Autodesk Inventor part; units mm, degrees
(part 3 of 4)
sketch "All Together" plane through (0, 0, 1.8) normal (0, 0, 1) x (1, 0, 0)
  arc A0 (70.625, 11.2735) -> (71.75, 14.25) centre (67.25, 14.25) ccw projected
  line L0 (71.75, 14.25) -> (71.75, 43.95) projected
  arc A1 (71.75, 43.95) -> (70.625, 46.9265) centre (67.25, 43.95) ccw projected
  arc A2 (70.1483, 47.7318) -> (70.625, 46.9265) centre (72.5, 48.5801) ccw projected
  arc A3 (70.1483, 47.7318) -> (69.436, 47.9997) centre (69.678, 47.5622) ccw projected
  arc A4 (63.9168, 53.2778) -> (69.436, 47.9997) centre (67.5, 51.5) ccw projected
  arc A5 (63.9168, 53.2778) -> (63.4689, 54) centre (63.4689, 53.5) ccw projected
  line L1 (63.4689, 54) -> (-63.4689, 54) projected
  arc A6 (-63.4689, 54) -> (-63.9168, 53.2778) centre (-63.4689, 53.5) ccw projected
  arc A7 (-69.2778, 47.9168) -> (-63.9168, 53.2778) centre (-67.5, 51.5) ccw projected
  arc A8 (-69.2778, 47.9168) -> (-70, 47.4689) centre (-69.5, 47.4689) ccw projected
  line L2 (-70, 47.4689) -> (-70, 22.5) projected
  line L3 (-70, 22.5) -> (-54, 22.5) projected
  arc A9 (-51.5, 20) -> (-54, 22.5) centre (-54, 20) ccw projected
  line L4 (-51.5, 20) -> (-51.5, 17.8589) projected
  arc A10 (-51.5, 17.8589) -> (-50.8913, 16.5323) centre (-49.75, 17.8589) ccw projected
  arc A11 (-53.5, 9.5) -> (-50.8913, 16.5323) centre (-53.5, 13.5) ccw projected
  line L5 (-53.5, 9.5) -> (-68.5, 9.5) projected
  arc A12 (-70.1109, 9.8387) -> (-68.5, 9.5) centre (-68.5, 13.5) ccw projected
  arc A13 (-70, 9.1411) -> (-70.1109, 9.8387) centre (-72.25, 9.1411) ccw projected
  line L6 (-70, 9.1411) -> (-70, 3.5) projected
  line L7 (-70, 3.5) -> (-52.9019, 3.5) projected
  line L8 (-52.9019, 3.5) -> (-51.3142, 0.75) projected
  arc A14 (-51.3142, -2.75) -> (-51.3142, 0.75) centre (-54.3453, -1) ccw projected
  line L9 (-51.3142, -2.75) -> (-52.9019, -5.5) projected
  line L10 (-52.9019, -5.5) -> (-70, -5.5) projected
  line L11 (-70, -5.5) -> (-70, -10.5) projected
  arc A15 (-70.1419, -11.4865) -> (-70, -10.5) centre (-73.5, -10.5) ccw projected
  arc A16 (-54.6724, -28.431) -> (-70.1419, -11.4865) centre (-63, -20.5) ccw projected
  arc A17 (-54.6724, -28.431) -> (-55.5, -30.5) centre (-52.5, -30.5) ccw projected
  line L12 (-55.5, -30.5) -> (-55.5, -32.5) projected
  arc A18 (-58, -35) -> (-55.5, -32.5) centre (-58, -32.5) ccw projected
  line L13 (-58, -35) -> (-70, -35) projected
  line L14 (-70, -35) -> (-70, -37) projected
  line L15 (-70, -37) -> (-56.4793, -37) projected
  line L16 (-56.4793, -37) -> (-55.1802, -39.25) projected
  arc A19 (-55.1802, -41.75) -> (-55.1802, -39.25) centre (-57.3453, -40.5) ccw projected
  line L17 (-55.1802, -41.75) -> (-56.4793, -44) projected
  line L18 (-56.4793, -44) -> (-70, -44) projected
  line L19 (-70, -44) -> (-70, -47.4689) projected
  arc A20 (-70, -47.4689) -> (-69.2778, -47.9168) centre (-69.5, -47.4689) ccw projected
  arc A21 (-63.9168, -53.2778) -> (-69.2778, -47.9168) centre (-67.5, -51.5) ccw projected
  arc A22 (-63.9168, -53.2778) -> (-63.4689, -54) centre (-63.4689, -53.5) ccw projected
  line L20 (-63.4689, -54) -> (-47.5, -54) projected
  line L21 (-47.5, -54) -> (-47.5, -50) projected
  arc A23 (-45, -47.5) -> (-47.5, -50) centre (-45, -50) ccw projected
  line L22 (-45, -47.5) -> (24, -47.5) projected
  arc A24 (26.5, -50) -> (24, -47.5) centre (24, -50) ccw projected
  line L23 (26.5, -50) -> (26.5, -54) projected
  line L24 (26.5, -54) -> (63.4689, -54) projected
  arc A25 (63.4689, -54) -> (63.9168, -53.2778) centre (63.4689, -53.5) ccw projected
  arc A26 (69.2778, -47.9168) -> (63.9168, -53.2778) centre (67.5, -51.5) ccw projected
  arc A27 (69.2778, -47.9168) -> (70, -47.4689) centre (69.5, -47.4689) ccw projected
  line L25 (70, -47.4689) -> (70, -44) projected
  line L26 (70, -44) -> (56.366, -44) projected
  line L27 (56.366, -44) -> (58.0981, -41) projected
  arc A28 (58.0981, -41) -> (58.0981, -40) centre (57.2321, -40.5) ccw projected
  line L28 (58.0981, -40) -> (56.366, -37) projected
  line L29 (56.366, -37) -> (70, -37) projected
  line L30 (70, -37) -> (70, -30.5) projected
  arc A29 (70.1419, -29.5135) -> (70, -30.5) centre (73.5, -30.5) ccw projected
  arc A30 (54.6724, -12.569) -> (70.1419, -29.5135) centre (63, -20.5) ccw projected
  arc A31 (54.6724, -12.569) -> (55.5, -10.5) centre (52.5, -10.5) ccw projected
  line L31 (55.5, -10.5) -> (55.5, -8.5) projected
  arc A32 (58, -6) -> (55.5, -8.5) centre (58, -8.5) ccw projected
  line L32 (58, -6) -> (70, -6) projected
  line L33 (70, -6) -> (70, 9.6199) projected
  arc A33 (70.625, 11.2735) -> (70, 9.6199) centre (72.5, 9.6199) ccw projected
  line L34 (36.5, -14.0193) -> (36.5, -6) projected
  arc A34 (47.5, -6) -> (36.5, -6) centre (42, -6) ccw projected
  line L35 (47.5, -6) -> (47.5, -14.0193) projected
  arc A35 (49.5, -24.5) -> (47.5, -14.0193) centre (42, -20.5) ccw projected
  line L36 (49.5, -24.5) -> (49.5, -33.5) projected
  arc A36 (47, -36) -> (49.5, -33.5) centre (47, -33.5) ccw projected
  line L37 (47, -36) -> (37, -36) projected
  arc A37 (34.5, -33.5) -> (37, -36) centre (37, -33.5) ccw projected
  line L38 (34.5, -33.5) -> (34.5, -24.5) projected
  arc A38 (34.3389, -16.8179) -> (34.5, -24.5) centre (42, -20.5) ccw projected
  arc A39 (28.6611, -16.8179) -> (34.3389, -16.8179) centre (31.5, -14) ccw projected
  arc A40 (26.5, -26.9807) -> (28.6611, -16.8179) centre (21, -20.5) ccw projected
  line L39 (26.5, -26.9807) -> (26.5, -33.5) projected
  arc A41 (24, -36) -> (26.5, -33.5) centre (24, -33.5) ccw projected
  line L40 (24, -36) -> (18, -36) projected
  arc A42 (15.5, -33.5) -> (18, -36) centre (18, -33.5) ccw projected
  line L41 (15.5, -33.5) -> (15.5, -26.9807) projected
  arc A43 (13.3389, -16.8179) -> (15.5, -26.9807) centre (21, -20.5) ccw projected
  arc A44 (7.6611, -16.8179) -> (13.3389, -16.8179) centre (10.5, -14) ccw projected
  arc A45 (5.5, -26.9807) -> (7.6611, -16.8179) centre (0, -20.5) ccw projected
  line L42 (5.5, -26.9807) -> (5.5, -33.5) projected
  arc A46 (3, -36) -> (5.5, -33.5) centre (3, -33.5) ccw projected
  line L43 (3, -36) -> (-3, -36) projected
  arc A47 (-5.5, -33.5) -> (-3, -36) centre (-3, -33.5) ccw projected
  line L44 (-5.5, -33.5) -> (-5.5, -26.9807) projected
  arc A48 (-7.6611, -16.8179) -> (-5.5, -26.9807) centre (0, -20.5) ccw projected
  arc A49 (-13.3389, -16.8179) -> (-7.6611, -16.8179) centre (-10.5, -14) ccw projected
  arc A50 (-15.5, -26.9807) -> (-13.3389, -16.8179) centre (-21, -20.5) ccw projected
  line L45 (-15.5, -26.9807) -> (-15.5, -33.5) projected
  arc A51 (-18, -36) -> (-15.5, -33.5) centre (-18, -33.5) ccw projected
  line L46 (-18, -36) -> (-24, -36) projected
  arc A52 (-26.5, -33.5) -> (-24, -36) centre (-24, -33.5) ccw projected
  line L47 (-26.5, -33.5) -> (-26.5, -26.9807) projected
  arc A53 (-28.6611, -16.8179) -> (-26.5, -26.9807) centre (-21, -20.5) ccw projected
  arc A54 (-34.3389, -16.8179) -> (-28.6611, -16.8179) centre (-31.5, -14) ccw projected
  arc A55 (-36.5, -26.9807) -> (-34.3389, -16.8179) centre (-42, -20.5) ccw projected
  line L48 (-36.5, -26.9807) -> (-36.5, -33.5) projected
  arc A56 (-39, -36) -> (-36.5, -33.5) centre (-39, -33.5) ccw projected
  line L49 (-39, -36) -> (-45, -36) projected
  arc A57 (-47.5, -33.5) -> (-45, -36) centre (-45, -33.5) ccw projected
  line L50 (-47.5, -33.5) -> (-47.5, -26.9807) projected
  arc A58 (-47.5, -14.0193) -> (-47.5, -26.9807) centre (-42, -20.5) ccw projected
  line L51 (-47.5, -14.0193) -> (-47.5, -6) projected
  arc A59 (-36.5, -6) -> (-47.5, -6) centre (-42, -6) ccw projected
  line L52 (-36.5, -6) -> (-36.5, -14.0193) projected
  arc A60 (-35.2881, -15.2846) -> (-36.5, -14.0193) centre (-42, -20.5) ccw projected
  arc A61 (-27.7119, -15.2846) -> (-35.2881, -15.2846) centre (-31.5, -14) ccw projected
  arc A62 (-26.5, -14.0193) -> (-27.7119, -15.2846) centre (-21, -20.5) ccw projected
  line L53 (-26.5, -14.0193) -> (-26.5, -6) projected
  arc A63 (-15.5, -6) -> (-26.5, -6) centre (-21, -6) ccw projected
  line L54 (-15.5, -6) -> (-15.5, -14.0193) projected
  arc A64 (-14.2881, -15.2846) -> (-15.5, -14.0193) centre (-21, -20.5) ccw projected
  arc A65 (-6.7119, -15.2846) -> (-14.2881, -15.2846) centre (-10.5, -14) ccw projected
  arc A66 (-5.5, -14.0193) -> (-6.7119, -15.2846) centre (0, -20.5) ccw projected
  line L55 (-5.5, -14.0193) -> (-5.5, -6) projected
  arc A67 (5.5, -6) -> (-5.5, -6) centre (0, -6) ccw projected
  line L56 (5.5, -6) -> (5.5, -14.0193) projected
  arc A68 (6.7119, -15.2846) -> (5.5, -14.0193) centre (0, -20.5) ccw projected
  arc A69 (14.2881, -15.2846) -> (6.7119, -15.2846) centre (10.5, -14) ccw projected
  arc A70 (15.5, -14.0193) -> (14.2881, -15.2846) centre (21, -20.5) ccw projected
  line L57 (15.5, -14.0193) -> (15.5, -6) projected
  arc A71 (26.5, -6) -> (15.5, -6) centre (21, -6) ccw projected
  line L58 (26.5, -6) -> (26.5, -14.0193) projected
  arc A72 (27.7119, -15.2846) -> (26.5, -14.0193) centre (21, -20.5) ccw projected
  arc A73 (35.2881, -15.2846) -> (27.7119, -15.2846) centre (31.5, -14) ccw projected
  arc A74 (36.5, -14.0193) -> (35.2881, -15.2846) centre (42, -20.5) ccw projected
  circle A75 centre (35.75, 14.25) radius 3 projected
  line L59 (71, 39.1) -> (71, 22.1) projected
  arc A76 (67.5, 18.6) -> (71, 22.1) centre (67.5, 22.1) ccw projected
  line L60 (67.5, 18.6) -> (35.5, 18.6) projected
  arc A77 (32, 22.1) -> (35.5, 18.6) centre (35.5, 22.1) ccw projected
  line L61 (32, 22.1) -> (32, 39.1) projected
  arc A78 (33.4964, 41.9698) -> (32, 39.1) centre (35.5, 39.1) ccw projected
  arc A79 (38.4291, 42.6) -> (33.4964, 41.9698) centre (35.75, 43.95) ccw projected
  line L62 (38.4291, 42.6) -> (64.5709, 42.6) projected
  arc A80 (69.5036, 41.9698) -> (64.5709, 42.6) centre (67.25, 43.95) ccw projected
  arc A81 (71, 39.1) -> (69.5036, 41.9698) centre (67.5, 39.1) ccw projected
  circle A82 centre (67.25, 14.25) radius 3 projected
  circle A83 centre (-31.5, -14) radius 3.5 projected
  circle A84 centre (-31.5, -14) radius 1.6 projected
  circle A85 centre (-10.5, -14) radius 3.5 projected
  circle A86 centre (-10.5, -14) radius 1.6 projected
  circle A87 centre (10.5, -14) radius 3.5 projected
  circle A88 centre (10.5, -14) radius 1.6 projected
  circle A89 centre (31.5, -14) radius 3.5 projected
  circle A90 centre (31.5, -14) radius 1.6 projected
  line L63 (16, -6) -> (16, -14.255) projected
  arc A91 (26, -14.255) -> (16, -14.255) centre (21, -20.5) ccw projected
  line L64 (26, -14.255) -> (26, -6) projected
  arc A92 (26, -6) -> (16, -6) centre (21, -6) ccw projected
  circle A93 centre (21, -6) radius 2.75 projected
  line L65 (26, -33.5) -> (26, -26.745) projected
  arc A94 (16, -26.745) -> (26, -26.745) centre (21, -20.5) ccw projected
  line L66 (16, -26.745) -> (16, -33.5) projected
  arc A95 (16, -33.5) -> (18, -35.5) centre (18, -33.5) ccw projected
  line L67 (18, -35.5) -> (24, -35.5) projected
  arc A96 (24, -35.5) -> (26, -33.5) centre (24, -33.5) ccw projected
  line L68 (5, -33.5) -> (5, -26.745) projected
  arc A97 (-5, -26.745) -> (5, -26.745) centre (0, -20.5) ccw projected
  line L69 (-5, -26.745) -> (-5, -33.5) projected
  arc A98 (-5, -33.5) -> (-3, -35.5) centre (-3, -33.5) ccw projected
  line L70 (-3, -35.5) -> (3, -35.5) projected
  arc A99 (3, -35.5) -> (5, -33.5) centre (3, -33.5) ccw projected
  line L71 (-16, -33.5) -> (-16, -26.745) projected
  arc A100 (-26, -26.745) -> (-16, -26.745) centre (-21, -20.5) ccw projected
  line L72 (-26, -26.745) -> (-26, -33.5) projected
  arc A101 (-26, -33.5) -> (-24, -35.5) centre (-24, -33.5) ccw projected
  line L73 (-24, -35.5) -> (-18, -35.5) projected
  arc A102 (-18, -35.5) -> (-16, -33.5) centre (-18, -33.5) ccw projected
  line L74 (-37, -33.5) -> (-37, -26.745) projected
  arc A103 (-47, -26.745) -> (-37, -26.745) centre (-42, -20.5) ccw projected
  line L75 (-47, -26.745) -> (-47, -33.5) projected
  arc A104 (-47, -33.5) -> (-45, -35.5) centre (-45, -33.5) ccw projected
  line L76 (-45, -35.5) -> (-39, -35.5) projected
  arc A105 (-39, -35.5) -> (-37, -33.5) centre (-39, -33.5) ccw projected
  line L77 (-47, -6) -> (-47, -14.255) projected
  arc A106 (-37, -14.255) -> (-47, -14.255) centre (-42, -20.5) ccw projected
  line L78 (-37, -14.255) -> (-37, -6) projected
  arc A107 (-37, -6) -> (-47, -6) centre (-42, -6) ccw projected
  circle A108 centre (-42, -6) radius 2.75 projected
  line L79 (-26, -6) -> (-26, -14.255) projected
  arc A109 (-16, -14.255) -> (-26, -14.255) centre (-21, -20.5) ccw projected
  line L80 (-16, -14.255) -> (-16, -6) projected
  arc A110 (-16, -6) -> (-26, -6) centre (-21, -6) ccw projected
  circle A111 centre (-21, -6) radius 2.75 projected
  line L81 (-5, -6) -> (-5, -14.255) projected
  arc A112 (5, -14.255) -> (-5, -14.255) centre (0, -20.5) ccw projected
  line L82 (5, -14.255) -> (5, -6) projected
  arc A113 (5, -6) -> (-5, -6) centre (0, -6) ccw projected
  circle A114 centre (0, -6) radius 2.75 projected
  line L83 (38, -6) -> (38, -13.5718) projected
  arc A115 (46, -13.5718) -> (38, -13.5718) centre (42, -20.5) ccw projected
  line L84 (46, -13.5718) -> (46, -6) projected
  arc A116 (46, -6) -> (38, -6) centre (42, -6) ccw projected
  circle A117 centre (42, -6) radius 2.75 projected
  line L85 (37.5, -30) -> (37.5, -27.1144) projected
  arc A118 (35, -24.373) -> (37.5, -27.1144) centre (42, -20.5) ccw projected
  line L86 (35, -33.5) -> (35, -24.373) projected
  arc A119 (35, -33.5) -> (37, -35.5) centre (37, -33.5) ccw projected
  line L87 (47, -35.5) -> (37, -35.5) projected
  arc A120 (47, -35.5) -> (49, -33.5) centre (47, -33.5) ccw projected
  line L88 (49, -24.373) -> (49, -33.5) projected
  arc A121 (46.5, -27.1144) -> (49, -24.373) centre (42, -20.5) ccw projected
  line L89 (46.5, -27.1144) -> (46.5, -30) projected
  line L90 (46.5, -30) -> (46, -30) projected
  line L91 (46, -30) -> (46, -27.4282) projected
  arc A122 (38, -27.4282) -> (46, -27.4282) centre (42, -20.5) ccw projected
  line L92 (38, -27.4282) -> (38, -30) projected
  line L93 (38, -30) -> (37.5, -30) projected
  arc A123 (46.5, -6) -> (37.5, -6) centre (42, -6) ccw projected
  line L94 (37.5, -13.8856) -> (37.5, -6) projected
  arc A124 (38, -13.5718) -> (37.5, -13.8856) centre (42, -20.5) ccw projected
  line L95 (38, -6) -> (38, -13.5718) projected
  arc A125 (46, -6) -> (38, -6) centre (42, -6) ccw projected
  line L96 (46, -13.5718) -> (46, -6) projected
  arc A126 (46.5, -13.8856) -> (46, -13.5718) centre (42, -20.5) ccw projected
  line L97 (46.5, -6) -> (46.5, -13.8856) projected
  circle A127 centre (63, -20.5) radius 8 projected
  arc A128 (70, -10.5) -> (70.9655, -12.9138) centre (73.5, -10.5) ccw projected
  line L98 (70, -6.5) -> (70, -10.5) projected
  line L99 (58, -6.5) -> (70, -6.5) projected
  arc A129 (58, -6.5) -> (56, -8.5) centre (58, -8.5) ccw projected
  line L100 (56, -10.5) -> (56, -8.5) projected
  arc A130 (55.0345, -12.9138) -> (56, -10.5) centre (52.5, -10.5) ccw projected
  arc A131 (55.0345, -12.9138) -> (70.9655, -12.9138) centre (63, -20.5) ccw projected
  line L101 (-70.5, -37.5) -> (-70.5, -30.5) projected
  arc A132 (-70.5, -30.5) -> (-71.3276, -28.431) centre (-73.5, -30.5) ccw projected
  arc A133 (-71.3276, -12.569) -> (-71.3276, -28.431) centre (-63, -20.5) ccw projected
  arc A134 (-71.3276, -12.569) -> (-70.5, -10.5) centre (-73.5, -10.5) ccw projected
  line L102 (-70.5, -10.5) -> (-70.5, -5) projected
  line L103 (-53.1906, -5) -> (-70.5, -5) projected
  line L104 (-51.7472, -2.5) -> (-53.1906, -5) projected
  arc A135 (-51.7472, -2.5) -> (-51.7472, 0.5) centre (-54.3453, -1) ccw projected
  line L105 (-53.1906, 3) -> (-51.7472, 0.5) projected
  line L106 (-70.5, 3) -> (-53.1906, 3) projected
  line L107 (-70.5, 3) -> (-70.5, 9.1411) projected
  arc A136 (-70.5, 9.1411) -> (-71.1087, 10.4677) centre (-72.25, 9.1411) ccw projected
  arc A137 (-71.1087, 16.5323) -> (-71.1087, 10.4677) centre (-68.5, 13.5) ccw projected
  arc A138 (-71.1087, 16.5323) -> (-70.5, 17.8589) centre (-72.25, 17.8589) ccw projected
  line L108 (-70.5, 17.8589) -> (-70.5, 47.4689) projected
  arc A139 (-69.0556, 48.3647) -> (-70.5, 47.4689) centre (-69.5, 47.4689) ccw projected
  arc A140 (-69.0556, 48.3647) -> (-64.3647, 53.0556) centre (-67.5, 51.5) ccw projected
  arc A141 (-63.4689, 54.5) -> (-64.3647, 53.0556) centre (-63.4689, 53.5) ccw projected
  line L109 (-63.4689, 54.5) -> (63.4689, 54.5) projected
  arc A142 (64.3647, 53.0556) -> (63.4689, 54.5) centre (63.4689, 53.5) ccw projected
  arc A143 (64.3647, 53.0556) -> (69.194, 48.4372) centre (67.5, 51.5) ccw projected
  arc A144 (70.6186, 47.9015) -> (69.194, 48.4372) centre (69.678, 47.5622) ccw projected
  arc A145 (70.6186, 47.9015) -> (71, 47.2572) centre (72.5, 48.5801) ccw projected
  arc A146 (72.25, 43.95) -> (71, 47.2572) centre (67.25, 43.95) ccw projected
  line L110 (72.25, 43.95) -> (72.25, 14.25) projected
  arc A147 (71, 10.9428) -> (72.25, 14.25) centre (67.25, 14.25) ccw projected
  arc A148 (71, 10.9428) -> (70.5, 9.6199) centre (72.5, 9.6199) ccw projected
  line L111 (70.5, 9.6199) -> (70.5, -10.5) projected
  arc A149 (70.5, -10.5) -> (71.3276, -12.569) centre (73.5, -10.5) ccw projected
  arc A150 (71.3276, -28.431) -> (71.3276, -12.569) centre (63, -20.5) ccw projected
  arc A151 (71.3276, -28.431) -> (70.5, -30.5) centre (73.5, -30.5) ccw projected
  line L112 (70.5, -30.5) -> (70.5, -37.5) projected
  line L113 (57.2321, -37.5) -> (70.5, -37.5) projected
  line L114 (58.5311, -39.75) -> (57.2321, -37.5) projected
  arc A152 (58.5311, -41.25) -> (58.5311, -39.75) centre (57.2321, -40.5) ccw projected
  line L115 (57.2321, -43.5) -> (58.5311, -41.25) projected
  line L116 (70.5, -43.5) -> (57.2321, -43.5) projected
  line L117 (70.5, -43.5) -> (70.5, -47.4689) projected
  arc A153 (69.0556, -48.3647) -> (70.5, -47.4689) centre (69.5, -47.4689) ccw projected
  arc A154 (69.0556, -48.3647) -> (64.3647, -53.0556) centre (67.5, -51.5) ccw projected
  arc A155 (63.4689, -54.5) -> (64.3647, -53.0556) centre (63.4689, -53.5) ccw projected
  line L118 (63.4689, -54.5) -> (26, -54.5) projected
  line L119 (26, -50) -> (26, -54.5) projected
  arc A156 (26, -50) -> (24, -48) centre (24, -50) ccw projected
  line L120 (-45, -48) -> (24, -48) projected
  arc A157 (-45, -48) -> (-47, -50) centre (-45, -50) ccw projected
  line L121 (-47, -54.5) -> (-47, -50) projected
  line L122 (-47, -54.5) -> (-63.4689, -54.5) projected
  arc A158 (-64.3647, -53.0556) -> (-63.4689, -54.5) centre (-63.4689, -53.5) ccw projected
  arc A159 (-64.3647, -53.0556) -> (-69.0556, -48.3647) centre (-67.5, -51.5) ccw projected
  arc A160 (-70.5, -47.4689) -> (-69.0556, -48.3647) centre (-69.5, -47.4689) ccw projected
  line L123 (-70.5, -47.4689) -> (-70.5, -43.5) projected
  line L124 (-56.7679, -43.5) -> (-70.5, -43.5) projected
  line L125 (-55.6132, -41.5) -> (-56.7679, -43.5) projected
  arc A161 (-55.6132, -41.5) -> (-55.6132, -39.5) centre (-57.3453, -40.5) ccw projected
  line L126 (-56.7679, -37.5) -> (-55.6132, -39.5) projected
  line L127 (-70.5, -37.5) -> (-56.7679, -37.5) projected
  line L128 (-70.5, -4.5) -> (-70.5, 2.5) projected
  line L129 (-53.4793, 2.5) -> (-70.5, 2.5) projected
  line L130 (-52.1802, 0.25) -> (-53.4793, 2.5) projected
  arc A162 (-52.1802, -2.25) -> (-52.1802, 0.25) centre (-54.3453, -1) ccw projected
  line L131 (-53.4793, -4.5) -> (-52.1802, -2.25) projected
  line L132 (-70.5, -4.5) -> (-53.4793, -4.5) projected
  line L133 (-57.0566, -38) -> (-70.5, -38) projected
  line L134 (-56.0463, -39.75) -> (-57.0566, -38) projected
  arc A163 (-56.0463, -41.25) -> (-56.0463, -39.75) centre (-57.3453, -40.5) ccw projected
  line L135 (-57.0566, -43) -> (-56.0463, -41.25) projected
  line L136 (-70.5, -43) -> (-57.0566, -43) projected
  line L137 (-70.5, -43) -> (-70.5, -38) projected
  line L138 (58.0981, -43) -> (70.5, -43) projected
  line L139 (58.9641, -41.5) -> (58.0981, -43) projected
  arc A164 (58.9641, -41.5) -> (58.9641, -39.5) centre (57.2321, -40.5) ccw projected
  line L140 (58.0981, -38) -> (58.9641, -39.5) projected
  line L141 (70.5, -38) -> (58.0981, -38) projected
  line L142 (70.5, -38) -> (70.5, -43) projected
  arc A165 (-71.4348, 16.9113) -> (-71, 17.8589) centre (-72.25, 17.8589) ccw projected
  arc A166 (-71.4348, 16.9113) -> (-71.4348, 10.0887) centre (-68.5, 13.5) ccw projected
  arc A167 (-71, 9.1411) -> (-71.4348, 10.0887) centre (-72.25, 9.1411) ccw projected
  line L143 (-71, 9.1411) -> (-71, -10.5) projected
  arc A168 (-71.6897, -12.2241) -> (-71, -10.5) centre (-73.5, -10.5) ccw projected
  arc A169 (-71.6897, -12.2241) -> (-71.6897, -28.7759) centre (-63, -20.5) ccw projected
  arc A170 (-71, -30.5) -> (-71.6897, -28.7759) centre (-73.5, -30.5) ccw projected
  line L144 (-71, -30.5) -> (-71, -51.5) projected
  arc A171 (-71, -51.5) -> (-67.5, -55) centre (-67.5, -51.5) ccw projected
  line L145 (-67.5, -55) -> (67.5, -55) projected
  arc A172 (67.5, -55) -> (71, -51.5) centre (67.5, -51.5) ccw projected
  line L146 (71, -51.5) -> (71, -30.5) projected
  arc A173 (71.6897, -28.7759) -> (71, -30.5) centre (73.5, -30.5) ccw projected
  arc A174 (71.6897, -28.7759) -> (71.6897, -12.2241) centre (63, -20.5) ccw projected
  arc A175 (71, -10.5) -> (71.6897, -12.2241) centre (73.5, -10.5) ccw projected
  line L147 (71, -10.5) -> (71, 9.6199) projected
  arc A176 (71.375, 10.6121) -> (71, 9.6199) centre (72.5, 9.6199) ccw projected
  arc A177 (71.375, 10.6121) -> (72.75, 14.25) centre (67.25, 14.25) ccw projected
  line L148 (72.75, 14.25) -> (72.75, 43.95) projected
  arc A178 (72.75, 43.95) -> (71.375, 47.5879) centre (67.25, 43.95) ccw projected
  arc A179 (71, 48.5801) -> (71.375, 47.5879) centre (72.5, 48.5801) ccw projected
  line L149 (71, 48.5801) -> (71, 51.5) projected
  arc A180 (71, 51.5) -> (67.5, 55) centre (67.5, 51.5) ccw projected
  line L150 (67.5, 55) -> (-67.5, 55) projected
  arc A181 (-67.5, 55) -> (-71, 51.5) centre (-67.5, 51.5) ccw projected
  line L151 (-71, 51.5) -> (-71, 17.8589) projected
  circle A182 centre (67.5, 51.5) radius 1.6 projected
  circle A183 centre (67.5, -51.5) radius 1.6 projected
  circle A184 centre (-67.5, -51.5) radius 1.6 projected
  circle A185 centre (-67.5, 51.5) radius 1.6 projected
  line L152 (-46.5, -50) -> (-46.5, -54.5) projected
  arc A186 (-45, -48.5) -> (-46.5, -50) centre (-45, -50) ccw projected
  line L153 (24, -48.5) -> (-45, -48.5) projected
  arc A187 (25.5, -50) -> (24, -48.5) centre (24, -50) ccw projected
  line L154 (25.5, -54.5) -> (25.5, -50) projected
  line L155 (25.5, -54.5) -> (-46.5, -54.5) projected
  circle A188 centre (-63, -20.5) radius 8 projected
  arc A189 (-70, -30.5) -> (-70.9655, -28.0862) centre (-73.5, -30.5) ccw projected
  line L156 (-70, -34.5) -> (-70, -30.5) projected
  line L157 (-58, -34.5) -> (-70, -34.5) projected
  arc A190 (-58, -34.5) -> (-56, -32.5) centre (-58, -32.5) ccw projected
  line L158 (-56, -30.5) -> (-56, -32.5) projected
  arc A191 (-55.0345, -28.0862) -> (-56, -30.5) centre (-52.5, -30.5) ccw projected
  arc A192 (-55.0345, -28.0862) -> (-70.9655, -28.0862) centre (-63, -20.5) ccw projected
  line L159 (33, 39.1) -> (33, 22.1) projected
  arc A193 (33.5215, 40.6283) -> (33, 39.1) centre (35.5, 39.1) ccw projected
  arc A194 (33.1245, 40.9322) -> (33.5215, 40.6283) centre (35.75, 43.95) ccw projected
  arc A195 (33.1245, 40.9322) -> (32.5, 39.1) centre (35.5, 39.1) ccw projected
  line L160 (32.5, 22.1) -> (32.5, 39.1) projected
  arc A196 (32.5, 22.1) -> (35.5, 19.1) centre (35.5, 22.1) ccw projected
  line L161 (67.5, 19.1) -> (35.5, 19.1) projected
  arc A197 (67.5, 19.1) -> (70.5, 22.1) centre (67.5, 22.1) ccw projected
  line L162 (70.5, 39.1) -> (70.5, 22.1) projected
  arc A198 (70.5, 39.1) -> (69.8755, 40.9322) centre (67.5, 39.1) ccw projected
  arc A199 (69.4785, 40.6283) -> (69.8755, 40.9322) centre (67.25, 43.95) ccw projected
  arc A200 (70, 39.1) -> (69.4785, 40.6283) centre (67.5, 39.1) ccw projected
  line L163 (70, 22.1) -> (70, 39.1) projected
  arc A201 (67.5, 19.6) -> (70, 22.1) centre (67.5, 22.1) ccw projected
  line L164 (35.5, 19.6) -> (67.5, 19.6) projected
  arc A202 (33, 22.1) -> (35.5, 19.6) centre (35.5, 22.1) ccw projected
  line L165 (69, 22.1) -> (69, 39.1) projected
  arc A203 (67.5, 20.6) -> (69, 22.1) centre (67.5, 22.1) ccw projected
  line L166 (35.5, 20.6) -> (67.5, 20.6) projected
  arc A204 (34, 22.1) -> (35.5, 20.6) centre (35.5, 22.1) ccw projected
  line L167 (34, 39.1) -> (34, 22.1) projected
  arc A205 (34.4469, 40.1682) -> (34, 39.1) centre (35.5, 39.1) ccw projected
  arc A206 (33.9581, 40.3738) -> (34.4469, 40.1682) centre (35.75, 43.95) ccw projected
  arc A207 (33.9581, 40.3738) -> (33.5, 39.1) centre (35.5, 39.1) ccw projected
  line L168 (33.5, 22.1) -> (33.5, 39.1) projected
  arc A208 (33.5, 22.1) -> (35.5, 20.1) centre (35.5, 22.1) ccw projected
  line L169 (67.5, 20.1) -> (35.5, 20.1) projected
  arc A209 (67.5, 20.1) -> (69.5, 22.1) centre (67.5, 22.1) ccw projected
  line L170 (69.5, 39.1) -> (69.5, 22.1) projected
  arc A210 (69.5, 39.1) -> (69.0419, 40.3738) centre (67.5, 39.1) ccw projected
  arc A211 (68.5531, 40.1682) -> (69.0419, 40.3738) centre (67.25, 43.95) ccw projected
  arc A212 (69, 39.1) -> (68.5531, 40.1682) centre (67.5, 39.1) ccw projected
  line L171 (39.2965, 42.1) -> (63.7035, 42.1) projected
  arc A213 (38.9869, 41.6) -> (39.2965, 42.1) centre (35.75, 43.95) ccw projected
  line L172 (64.0131, 41.6) -> (38.9869, 41.6) projected
  arc A214 (63.7035, 42.1) -> (64.0131, 41.6) centre (67.25, 43.95) ccw projected
  arc A215 (64.4433, 41.1) -> (65.0643, 40.6) centre (67.25, 43.95) ccw projected
  line L173 (38.5567, 41.1) -> (64.4433, 41.1) projected
  arc A216 (37.9357, 40.6) -> (38.5567, 41.1) centre (35.75, 43.95) ccw projected
  line L174 (65.0643, 40.6) -> (37.9357, 40.6) projected
  circle A217 centre (35.75, 14.25) radius 3 projected
  circle A218 centre (67.25, 14.25) radius 3 projected
  circle A219 centre (67.25, 43.95) radius 3 projected
  circle A220 centre (35.75, 43.95) radius 3 projected
  line L175 (34.5, 39.1) -> (34.5, 22.1) projected
  arc A221 (34.5, 22.1) -> (35.5, 21.1) centre (35.5, 22.1) ccw projected
  line L176 (35.5, 21.1) -> (67.5, 21.1) projected
  arc A222 (67.5, 21.1) -> (68.5, 22.1) centre (67.5, 22.1) ccw projected
  line L177 (68.5, 22.1) -> (68.5, 39.1) projected
  arc A223 (68.5, 39.1) -> (67.5, 40.1) centre (67.5, 39.1) ccw projected
  line L178 (67.5, 40.1) -> (35.5, 40.1) projected
  arc A224 (35.5, 40.1) -> (34.5, 39.1) centre (35.5, 39.1) ccw projected
  circle A225 centre (-53.5, 13.5) radius 1.7 projected
  circle A226 centre (-58.5, 13.5) radius 1.7 projected
  circle A227 centre (-63.5, 13.5) radius 1.7 projected
  circle A228 centre (-68.5, 13.5) radius 1.7 projected
  circle A229 centre (42, -6) radius 2.75 projected
  circle A230 centre (21, -6) radius 2.75 projected
  circle A231 centre (0, -6) radius 2.75 projected
  circle A232 centre (-21, -6) radius 2.75 projected
  circle A233 centre (-42, -6) radius 2.75 projected
  circle A234 centre (63, -20.5) radius 8 projected
  circle A235 centre (42, -20.5) radius 8 projected
  circle A236 centre (21, -20.5) radius 8 projected
  circle A237 centre (0, -20.5) radius 8 projected
  circle A238 centre (-21, -20.5) radius 8 projected
  circle A239 centre (-42, -20.5) radius 8 projected
  circle A240 centre (-63, -20.5) radius 8 projected
  circle A241 centre (-67.5, -51.5) radius 1.6 projected
  circle A242 centre (67.5, -51.5) radius 1.6 projected
  circle A243 centre (67.5, 51.5) radius 1.6 projected
  circle A244 centre (-67.5, 51.5) radius 1.6 projected
  circle A245 centre (10.5, -14) radius 1.6 projected
  circle A246 centre (-10.5, -14) radius 1.6 projected
  circle A247 centre (31.5, -14) radius 1.6 projected
  circle A248 centre (-31.5, -14) radius 1.6 projected
  arc A249 (67.5, -55.5) -> (71.5, -51.5) centre (67.5, -51.5) ccw projected
  line L179 (-67.5, -55.5) -> (67.5, -55.5) projected
  arc A250 (-71.5, -51.5) -> (-67.5, -55.5) centre (-67.5, -51.5) ccw projected
  line L180 (-71.5, -30.5) -> (-71.5, -51.5) projected
  arc A251 (-71.5, -30.5) -> (-72.0517, -29.1207) centre (-73.5, -30.5) ccw projected
  arc A252 (-72.0517, -11.8793) -> (-72.0517, -29.1207) centre (-63, -20.5) ccw projected
  arc A253 (-72.0517, -11.8793) -> (-71.5, -10.5) centre (-73.5, -10.5) ccw projected
  line L181 (-71.5, 9.1411) -> (-71.5, -10.5) projected
  arc A254 (-71.5, 9.1411) -> (-71.7609, 9.7097) centre (-72.25, 9.1411) ccw projected
  arc A255 (-71.7609, 17.2903) -> (-71.7609, 9.7097) centre (-68.5, 13.5) ccw projected
  arc A256 (-71.7609, 17.2903) -> (-71.5, 17.8589) centre (-72.25, 17.8589) ccw projected
  line L182 (-71.5, 51.5) -> (-71.5, 17.8589) projected
  arc A257 (-67.5, 55.5) -> (-71.5, 51.5) centre (-67.5, 51.5) ccw projected
  line L183 (67.5, 55.5) -> (-67.5, 55.5) projected
  arc A258 (71.5, 51.5) -> (67.5, 55.5) centre (67.5, 51.5) ccw projected
  line L184 (71.5, 48.5801) -> (71.5, 51.5) projected
  arc A259 (71.5, 48.5801) -> (71.75, 47.9186) centre (72.5, 48.5801) ccw projected
  arc A260 (73.25, 43.95) -> (71.75, 47.9186) centre (67.25, 43.95) ccw projected
  line L185 (73.25, 43.95) -> (73.25, 14.25) projected
  arc A261 (71.75, 10.2814) -> (73.25, 14.25) centre (67.25, 14.25) ccw projected
  arc A262 (71.75, 10.2814) -> (71.5, 9.6199) centre (72.5, 9.6199) ccw projected
  line L186 (71.5, -10.5) -> (71.5, 9.6199) projected
  arc A263 (71.5, -10.5) -> (72.0517, -11.8793) centre (73.5, -10.5) ccw projected
  arc A264 (72.0517, -29.1207) -> (72.0517, -11.8793) centre (63, -20.5) ccw projected
  arc A265 (72.0517, -29.1207) -> (71.5, -30.5) centre (73.5, -30.5) ccw projected
  line L187 (71.5, -51.5) -> (71.5, -30.5) projected
  line L188 (37, -14.255) -> (37, -6) projected
  line L189 (37.5, -13.8856) -> (37.5, -6) projected
  arc A266 (46.5, -6) -> (37.5, -6) centre (42, -6) ccw projected
  line L190 (46.5, -6) -> (46.5, -13.8856) projected
  arc A267 (47, -14.255) -> (46.5, -13.8856) centre (42, -20.5) ccw projected
  line L191 (47, -6) -> (47, -14.255) projected
  arc A268 (47, -6) -> (37, -6) centre (42, -6) ccw projected
  line L192 (37, -14.255) -> (37, -6) projected
  arc A269 (37.5, -13.8856) -> (37, -14.255) centre (42, -20.5) ccw projected
  arc A270 (37.5, -27.1144) -> (38, -27.4282) centre (42, -20.5) ccw projected
  line L193 (37.5, -30) -> (37.5, -27.1144) projected
  line L194 (38, -30) -> (37.5, -30) projected
  line L195 (38, -27.4282) -> (38, -30) projected
  arc A271 (46, -27.4282) -> (46.5, -27.1144) centre (42, -20.5) ccw projected
  line L196 (46, -30) -> (46, -27.4282) projected
  line L197 (46.5, -30) -> (46, -30) projected
  line L198 (46.5, -27.1144) -> (46.5, -30) projected
  line L199 (-70, 22) -> (-54, 22) projected
  line L200 (-70, 17.8589) -> (-70, 22) projected
  arc A272 (-70.7826, 16.1532) -> (-70, 17.8589) centre (-72.25, 17.8589) ccw projected
  arc A273 (-70.7826, 16.1532) -> (-68.5, 10) centre (-68.5, 13.5) ccw projected
  line L201 (-53.5, 10) -> (-68.5, 10) projected
  arc A274 (-53.5, 10) -> (-51.2174, 16.1532) centre (-53.5, 13.5) ccw projected
  arc A275 (-52, 17.8589) -> (-51.2174, 16.1532) centre (-49.75, 17.8589) ccw projected
  line L202 (-52, 20) -> (-52, 17.8589) projected
  arc A276 (-52, 20) -> (-54, 22) centre (-54, 20) ccw projected
  circle A277 centre (-68.5, 13.5) radius 1.7 projected
  circle A278 centre (-53.5, 13.5) radius 1.7 projected
  circle A279 centre (-58.5, 13.5) radius 1.7 projected
  circle A280 centre (-63.5, 13.5) radius 1.7 projected
  point P0 (0, 0)
  constraints: 1 other
sketch "Sketch21" plane through (0, 0, 1.6) normal (0, 0, 1) x (1, 0, 0)
  line L0 (33.5, 22.1) -> (33.5, 39.1) projected
  arc A0 (33.9581, 40.3738) -> (33.5, 39.1) centre (35.5, 39.1) ccw projected
  arc A1 (33.9581, 40.3738) -> (34.4469, 40.1682) centre (35.75, 43.95) ccw projected
  arc A2 (34.4469, 40.1682) -> (34, 39.1) centre (35.5, 39.1) ccw projected
  line L1 (34, 39.1) -> (34, 22.1) projected
  arc A3 (34, 22.1) -> (35.5, 20.6) centre (35.5, 22.1) ccw projected
  line L2 (35.5, 20.6) -> (67.5, 20.6) projected
  arc A4 (67.5, 20.6) -> (69, 22.1) centre (67.5, 22.1) ccw projected
  line L3 (69, 22.1) -> (69, 39.1) projected
  arc A5 (69, 39.1) -> (68.5531, 40.1682) centre (67.5, 39.1) ccw projected
  arc A6 (68.5531, 40.1682) -> (69.0419, 40.3738) centre (67.25, 43.95) ccw projected
  arc A7 (69.5, 39.1) -> (69.0419, 40.3738) centre (67.5, 39.1) ccw projected
  line L4 (69.5, 39.1) -> (69.5, 22.1) projected
  arc A8 (67.5, 20.1) -> (69.5, 22.1) centre (67.5, 22.1) ccw projected
  line L5 (67.5, 20.1) -> (35.5, 20.1) projected
  arc A9 (33.5, 22.1) -> (35.5, 20.1) centre (35.5, 22.1) ccw projected
  arc A10 (70.5, 39.1) -> (69.8755, 40.9322) centre (67.5, 39.1) ccw projected
  line L6 (70.5, 39.1) -> (70.5, 22.1) projected
  arc A11 (67.5, 19.1) -> (70.5, 22.1) centre (67.5, 22.1) ccw projected
  line L7 (67.5, 19.1) -> (35.5, 19.1) projected
  arc A12 (32.5, 22.1) -> (35.5, 19.1) centre (35.5, 22.1) ccw projected
  line L8 (32.5, 22.1) -> (32.5, 39.1) projected
  arc A13 (33.1245, 40.9322) -> (32.5, 39.1) centre (35.5, 39.1) ccw projected
  arc A14 (33.1245, 40.9322) -> (33.5215, 40.6283) centre (35.75, 43.95) ccw projected
  arc A15 (33.5215, 40.6283) -> (33, 39.1) centre (35.5, 39.1) ccw projected
  line L9 (33, 39.1) -> (33, 22.1) projected
  arc A16 (33, 22.1) -> (35.5, 19.6) centre (35.5, 22.1) ccw projected
  line L10 (35.5, 19.6) -> (67.5, 19.6) projected
  arc A17 (67.5, 19.6) -> (70, 22.1) centre (67.5, 22.1) ccw projected
  line L11 (70, 22.1) -> (70, 39.1) projected
  arc A18 (70, 39.1) -> (69.4785, 40.6283) centre (67.5, 39.1) ccw projected
  arc A19 (69.4785, 40.6283) -> (69.8755, 40.9322) centre (67.25, 43.95) ccw projected
  arc A20 (37.9357, 40.6) -> (38.5567, 41.1) centre (35.75, 43.95) ccw projected
  line L12 (38.5567, 41.1) -> (64.4433, 41.1) projected
  arc A21 (64.4433, 41.1) -> (65.0643, 40.6) centre (67.25, 43.95) ccw projected
  line L13 (65.0643, 40.6) -> (37.9357, 40.6) projected
  arc A22 (63.7035, 42.1) -> (64.0131, 41.6) centre (67.25, 43.95) ccw projected
  line L14 (64.0131, 41.6) -> (38.9869, 41.6) projected
  arc A23 (38.9869, 41.6) -> (39.2965, 42.1) centre (35.75, 43.95) ccw projected
  line L15 (39.2965, 42.1) -> (63.7035, 42.1) projected
  line L16 (49, -24.373) -> (49, -33.5) projected
  arc A24 (47, -35.5) -> (49, -33.5) centre (47, -33.5) ccw projected
  line L17 (47, -35.5) -> (37, -35.5) projected
  arc A25 (35, -33.5) -> (37, -35.5) centre (37, -33.5) ccw projected
  line L18 (35, -33.5) -> (35, -24.373) projected
  arc A26 (37, -14.255) -> (35, -24.373) centre (42, -20.5) ccw projected
  line L19 (37, -14.255) -> (37, -6) projected
  arc A27 (47, -6) -> (37, -6) centre (42, -6) ccw projected
  line L20 (47, -6) -> (47, -14.255) projected
  arc A28 (49, -24.373) -> (47, -14.255) centre (42, -20.5) ccw projected
  line L21 (34.5, 22.1) -> (34.5, 39.1) projected
  arc A29 (35.5, 40.1) -> (34.5, 39.1) centre (35.5, 39.1) ccw projected
  line L22 (35.5, 40.1) -> (67.5, 40.1) projected
  arc A30 (68.5, 39.1) -> (67.5, 40.1) centre (67.5, 39.1) ccw projected
  line L23 (68.5, 39.1) -> (68.5, 22.1) projected
  arc A31 (67.5, 21.1) -> (68.5, 22.1) centre (67.5, 22.1) ccw projected
  line L24 (67.5, 21.1) -> (35.5, 21.1) projected
  arc A32 (34.5, 22.1) -> (35.5, 21.1) centre (35.5, 22.1) ccw projected
  circle A33 centre (35.75, 43.95) radius 3 projected
  circle A34 centre (67.25, 43.95) radius 3 projected
  circle A35 centre (67.25, 14.25) radius 3 projected
  circle A36 centre (35.75, 14.25) radius 3 projected
  circle A37 centre (-31.5, -14) radius 3.5 projected
  circle A38 centre (31.5, -14) radius 3.5 projected
  circle A39 centre (-10.5, -14) radius 3.5 projected
  circle A40 centre (10.5, -14) radius 3.5 projected
  line L25 (-47, -33.5) -> (-47, -26.745) projected
  arc A41 (-47, -14.255) -> (-47, -26.745) centre (-42, -20.5) ccw projected
  line L26 (-47, -14.255) -> (-47, -6) projected
  arc A42 (-37, -6) -> (-47, -6) centre (-42, -6) ccw projected
  line L27 (-37, -6) -> (-37, -14.255) projected
  arc A43 (-37, -26.745) -> (-37, -14.255) centre (-42, -20.5) ccw projected
  line L28 (-37, -26.745) -> (-37, -33.5) projected
  arc A44 (-39, -35.5) -> (-37, -33.5) centre (-39, -33.5) ccw projected
  line L29 (-39, -35.5) -> (-45, -35.5) projected
  arc A45 (-47, -33.5) -> (-45, -35.5) centre (-45, -33.5) ccw projected
  line L30 (-26, -33.5) -> (-26, -26.745) projected
  arc A46 (-26, -14.255) -> (-26, -26.745) centre (-21, -20.5) ccw projected
  line L31 (-26, -14.255) -> (-26, -6) projected
  arc A47 (-16, -6) -> (-26, -6) centre (-21, -6) ccw projected
  line L32 (-16, -6) -> (-16, -14.255) projected
  arc A48 (-16, -26.745) -> (-16, -14.255) centre (-21, -20.5) ccw projected
  line L33 (-16, -26.745) -> (-16, -33.5) projected
  arc A49 (-18, -35.5) -> (-16, -33.5) centre (-18, -33.5) ccw projected
  line L34 (-18, -35.5) -> (-24, -35.5) projected
  arc A50 (-26, -33.5) -> (-24, -35.5) centre (-24, -33.5) ccw projected
  line L35 (-5, -33.5) -> (-5, -26.745) projected
  arc A51 (-5, -14.255) -> (-5, -26.745) centre (0, -20.5) ccw projected
  line L36 (-5, -14.255) -> (-5, -6) projected
  arc A52 (5, -6) -> (-5, -6) centre (0, -6) ccw projected
  line L37 (5, -6) -> (5, -14.255) projected
  arc A53 (5, -26.745) -> (5, -14.255) centre (0, -20.5) ccw projected
  line L38 (5, -26.745) -> (5, -33.5) projected
  arc A54 (3, -35.5) -> (5, -33.5) centre (3, -33.5) ccw projected
  line L39 (3, -35.5) -> (-3, -35.5) projected
  arc A55 (-5, -33.5) -> (-3, -35.5) centre (-3, -33.5) ccw projected
  line L40 (16, -33.5) -> (16, -26.745) projected
  arc A56 (16, -14.255) -> (16, -26.745) centre (21, -20.5) ccw projected
  line L41 (16, -14.255) -> (16, -6) projected
  arc A57 (26, -6) -> (16, -6) centre (21, -6) ccw projected
  line L42 (26, -6) -> (26, -14.255) projected
  arc A58 (26, -26.745) -> (26, -14.255) centre (21, -20.5) ccw projected
  line L43 (26, -26.745) -> (26, -33.5) projected
  arc A59 (24, -35.5) -> (26, -33.5) centre (24, -33.5) ccw projected
  line L44 (24, -35.5) -> (18, -35.5) projected
  arc A60 (16, -33.5) -> (18, -35.5) centre (18, -33.5) ccw projected
  arc A61 (58, -6.5) -> (56, -8.5) centre (58, -8.5) ccw projected
  line L45 (58, -6.5) -> (70, -6.5) projected
  line L46 (70, -6.5) -> (70, -10.5) projected
  arc A62 (70, -10.5) -> (70.9655, -12.9138) centre (73.5, -10.5) ccw projected
  arc A63 (55.0345, -12.9138) -> (70.9655, -12.9138) centre (63, -20.5) ccw projected
  arc A64 (55.0345, -12.9138) -> (56, -10.5) centre (52.5, -10.5) ccw projected
  line L47 (56, -10.5) -> (56, -8.5) projected
  arc A65 (-58, -34.5) -> (-56, -32.5) centre (-58, -32.5) ccw projected
  line L48 (-58, -34.5) -> (-70, -34.5) projected
  line L49 (-70, -34.5) -> (-70, -30.5) projected
  arc A66 (-70, -30.5) -> (-70.9655, -28.0862) centre (-73.5, -30.5) ccw projected
  arc A67 (-55.0345, -28.0862) -> (-70.9655, -28.0862) centre (-63, -20.5) ccw projected
  arc A68 (-55.0345, -28.0862) -> (-56, -30.5) centre (-52.5, -30.5) ccw projected
  line L50 (-56, -30.5) -> (-56, -32.5) projected
  line L51 (-53.5, 10) -> (-68.5, 10) projected
  arc A69 (-70.7826, 16.1532) -> (-68.5, 10) centre (-68.5, 13.5) ccw projected
  arc A70 (-70.7826, 16.1532) -> (-70, 17.8589) centre (-72.25, 17.8589) ccw projected
  line L52 (-70, 17.8589) -> (-70, 22) projected
  line L53 (-70, 22) -> (-54, 22) projected
  arc A71 (-52, 20) -> (-54, 22) centre (-54, 20) ccw projected
  line L54 (-52, 20) -> (-52, 17.8589) projected
  arc A72 (-52, 17.8589) -> (-51.2174, 16.1532) centre (-49.75, 17.8589) ccw projected
  arc A73 (-53.5, 10) -> (-51.2174, 16.1532) centre (-53.5, 13.5) ccw projected
  line L55 (-70.5, -37.5) -> (-56.7679, -37.5) projected
  line L56 (-56.7679, -37.5) -> (-55.6132, -39.5) projected
  arc A74 (-55.6132, -41.5) -> (-55.6132, -39.5) centre (-57.3453, -40.5) ccw projected
  line L57 (-55.6132, -41.5) -> (-56.7679, -43.5) projected
  line L58 (-56.7679, -43.5) -> (-70.5, -43.5) projected
  line L59 (-70.5, -43.5) -> (-70.5, -47.4689) projected
  arc A75 (-70.5, -47.4689) -> (-69.0556, -48.3647) centre (-69.5, -47.4689) ccw projected
  arc A76 (-64.3647, -53.0556) -> (-69.0556, -48.3647) centre (-67.5, -51.5) ccw projected
  arc A77 (-64.3647, -53.0556) -> (-63.4689, -54.5) centre (-63.4689, -53.5) ccw projected
  line L60 (-63.4689, -54.5) -> (-47, -54.5) projected
  line L61 (-47, -54.5) -> (-47, -50) projected
  arc A78 (-45, -48) -> (-47, -50) centre (-45, -50) ccw projected
  line L62 (-45, -48) -> (24, -48) projected
  arc A79 (26, -50) -> (24, -48) centre (24, -50) ccw projected
  line L63 (26, -50) -> (26, -54.5) projected
  line L64 (26, -54.5) -> (63.4689, -54.5) projected
  arc A80 (63.4689, -54.5) -> (64.3647, -53.0556) centre (63.4689, -53.5) ccw projected
  arc A81 (69.0556, -48.3647) -> (64.3647, -53.0556) centre (67.5, -51.5) ccw projected
  arc A82 (69.0556, -48.3647) -> (70.5, -47.4689) centre (69.5, -47.4689) ccw projected
  line L65 (70.5, -47.4689) -> (70.5, -43.5) projected
  line L66 (70.5, -43.5) -> (57.2321, -43.5) projected
  line L67 (57.2321, -43.5) -> (58.5311, -41.25) projected
  arc A83 (58.5311, -41.25) -> (58.5311, -39.75) centre (57.2321, -40.5) ccw projected
  line L68 (58.5311, -39.75) -> (57.2321, -37.5) projected
  line L69 (57.2321, -37.5) -> (70.5, -37.5) projected
  line L70 (70.5, -37.5) -> (70.5, -30.5) projected
  arc A84 (71.3276, -28.431) -> (70.5, -30.5) centre (73.5, -30.5) ccw projected
  arc A85 (71.3276, -28.431) -> (71.3276, -12.569) centre (63, -20.5) ccw projected
  arc A86 (70.5, -10.5) -> (71.3276, -12.569) centre (73.5, -10.5) ccw projected
  line L71 (70.5, -10.5) -> (70.5, 9.6199) projected
  arc A87 (71, 10.9428) -> (70.5, 9.6199) centre (72.5, 9.6199) ccw projected
  arc A88 (71, 10.9428) -> (72.25, 14.25) centre (67.25, 14.25) ccw projected
  line L72 (72.25, 14.25) -> (72.25, 43.95) projected
  arc A89 (72.25, 43.95) -> (71, 47.2572) centre (67.25, 43.95) ccw projected
  arc A90 (70.6186, 47.9015) -> (71, 47.2572) centre (72.5, 48.5801) ccw projected
  arc A91 (70.6186, 47.9015) -> (69.194, 48.4372) centre (69.678, 47.5622) ccw projected
  arc A92 (64.3647, 53.0556) -> (69.194, 48.4372) centre (67.5, 51.5) ccw projected
  arc A93 (64.3647, 53.0556) -> (63.4689, 54.5) centre (63.4689, 53.5) ccw projected
  line L73 (63.4689, 54.5) -> (-63.4689, 54.5) projected
  arc A94 (-63.4689, 54.5) -> (-64.3647, 53.0556) centre (-63.4689, 53.5) ccw projected
  arc A95 (-69.0556, 48.3647) -> (-64.3647, 53.0556) centre (-67.5, 51.5) ccw projected
  arc A96 (-69.0556, 48.3647) -> (-70.5, 47.4689) centre (-69.5, 47.4689) ccw projected
  line L74 (-70.5, 47.4689) -> (-70.5, 17.8589) projected
  arc A97 (-71.1087, 16.5323) -> (-70.5, 17.8589) centre (-72.25, 17.8589) ccw projected
  arc A98 (-71.1087, 16.5323) -> (-71.1087, 10.4677) centre (-68.5, 13.5) ccw projected
  arc A99 (-70.5, 9.1411) -> (-71.1087, 10.4677) centre (-72.25, 9.1411) ccw projected
  line L75 (-70.5, 9.1411) -> (-70.5, 3) projected
  line L76 (-70.5, 3) -> (-53.1906, 3) projected
  line L77 (-53.1906, 3) -> (-51.7472, 0.5) projected
  arc A100 (-51.7472, -2.5) -> (-51.7472, 0.5) centre (-54.3453, -1) ccw projected
  line L78 (-51.7472, -2.5) -> (-53.1906, -5) projected
  line L79 (-53.1906, -5) -> (-70.5, -5) projected
  line L80 (-70.5, -5) -> (-70.5, -10.5) projected
  arc A101 (-71.3276, -12.569) -> (-70.5, -10.5) centre (-73.5, -10.5) ccw projected
  arc A102 (-71.3276, -12.569) -> (-71.3276, -28.431) centre (-63, -20.5) ccw projected
  arc A103 (-70.5, -30.5) -> (-71.3276, -28.431) centre (-73.5, -30.5) ccw projected
  line L81 (-70.5, -30.5) -> (-70.5, -37.5) projected
  line L82 (-70.5, 36.5) -> (-10.5, 36.5) construction
  line L83 (-70.5, 33.5) -> (-10.5, 33.5)
  line L84 (-10.5, 39.5) -> (-70.5, 39.5)
  arc A104 (-70.5, 39.5) -> (-70.5, 33.5) centre (-70.5, 36.5) ccw
  arc A105 (-10.5, 33.5) -> (-10.5, 39.5) centre (-10.5, 36.5) ccw
  point P0 (0, 0)
  point P1 (-40.5, 36.5)
  dimension "d175" = 6
  dimension "d176" = 60
  dimension "d177" = 18
  constraints: 8 end point, 4 point on circle, 4 tangent, 2 centre point, 1 midpoint, 1 parallel, 1 perpendicular, 1 point on line
  measures "d175" distance between parallel lines of L83 L84
  measures "d176" distance of L82.start L82.end
  measures "d177" distance between parallel lines of L73 L82